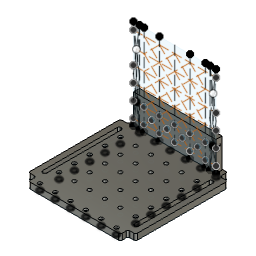
Whole_v2 v3 (Autodesk Fusion 360 design; units mm, degrees)
Autodesk Fusion 360 part; units mm, degrees
(part 1 of 2)
sketch "Sketch1" plane through (0, 0, 0) normal (0, 0, 1) x (1, 0, 0)
  line L0 (73.2, -88.9) -> (-73.2, -88.9)
  line L1 (-88.9, -73.2) -> (-88.9, 73.2)
  line L2 (-73.2, 88.9) -> (73.2, 88.9)
  line L3 (88.9, 73.2) -> (88.9, -73.2)
  line L4 (88.9, -88.9) -> (-88.9, 88.9) construction
  line L5 (-88.9, -88.9) -> (88.9, 88.9) construction
  line L6 (-88.9, 76.2) -> (88.9, 76.2) construction
  line L7 (-88.9, -76.2) -> (88.9, -76.2) construction
  line L8 (-76.2, 88.9) -> (-76.2, -88.9) construction
  line L9 (76.2, 88.9) -> (76.2, -88.9) construction
  line L10 (-76.2, 85.9) -> (-76.2, 79.2)
  line L11 (-85.9, 76.2) -> (-79.2, 76.2)
  line L12 (76.2, 85.9) -> (76.2, 79.2)
  line L13 (79.2, 76.2) -> (85.9, 76.2)
  line L14 (76.2, -76.2) -> (85.9, -76.2)
  line L15 (76.2, -85.9) -> (76.2, -79.2)
  line L16 (-76.2, -85.9) -> (-76.2, -79.2)
  line L17 (-85.9, -76.2) -> (-79.2, -76.2)
  line L18 (-75.85, -65) -> (-76.55, -65)
  line L19 (-79.55, -62) -> (-79.55, 62)
  line L20 (-76.3914, 65) -> (-75.85, 65)
  line L21 (-72.85, 62) -> (-72.85, -62)
  line L22 (-72.85, -65) -> (-79.3874, 61.8456) construction
  line L23 (-79.55, -65) -> (-72.85, 65) construction
  line L24 (76.55, -65) -> (75.85, -65)
  line L25 (72.85, -62) -> (72.85, 62)
  line L26 (75.85, 65) -> (76.55, 65)
  line L27 (79.55, 62) -> (79.55, -62)
  line L28 (79.55, -65) -> (72.85, 65) construction
  line L29 (72.85, -65) -> (79.55, 65) construction
  line L30 (-88.9, 82.55) -> (88.9, 82.55) construction
  line L31 (-63.5, 88.9) -> (-63.5, -88.9) construction
  line L32 (-38.1, 88.9) -> (-38.1, -88.9) construction
  line L33 (-12.7, 88.9) -> (-12.7, -88.9) construction
  line L34 (12.7, 88.9) -> (12.7, -88.9) construction
  line L35 (38.1, 88.9) -> (38.1, -88.9) construction
  line L36 (63.5, 88.9) -> (63.5, -88.9) construction
  line L37 (-88.9, -82.55) -> (88.9, -82.55) construction
  circle A0 centre (-63.5, 82.55) radius 3.1375
  circle A1 centre (-38.1, 82.55) radius 3.1375
  circle A2 centre (-12.7, 82.55) radius 3.1375
  circle A3 centre (12.7, 82.55) radius 3.1375
  circle A4 centre (38.1, 82.55) radius 3.1375
  circle A5 centre (63.5, 82.55) radius 3.1375
  line L38 (-88.9, 0) -> (88.9, 0) construction
  line L39 (-88.9, 50.8) -> (88.9, 50.8) construction
  line L40 (-88.9, 25.4) -> (88.9, 25.4) construction
  line L41 (-88.9, 0) -> (88.9, 0) construction
  line L42 (-88.9, -25.4) -> (88.9, -25.4) construction
  line L43 (-88.9, -50.8) -> (88.9, -50.8) construction
  line L44 (79.2, -76.2) -> (88.9, -76.2) construction
  circle A6 centre (-63.5, -82.55) radius 3.1375
  circle A7 centre (-38.1, -82.55) radius 3.1375
  circle A8 centre (-12.7, -82.55) radius 3.1375
  circle A9 centre (12.7, -82.55) radius 3.1375
  circle A10 centre (38.1, -82.55) radius 3.1375
  circle A11 centre (63.5, -82.55) radius 3.1375
  circle A12 centre (-63.5, 50.8) radius 3.1375
  circle A13 centre (-38.1, 50.8) radius 3.1375
  circle A14 centre (-12.7, 50.8) radius 3.1375
  circle A15 centre (12.7, 50.8) radius 3.1375
  circle A16 centre (38.1, 50.8) radius 3.1375
  circle A17 centre (63.5, 50.8) radius 3.1375
  circle A18 centre (-63.5, 25.4) radius 3.1375
  circle A19 centre (-38.1, 25.4) radius 3.1375
  circle A20 centre (-12.7, 25.4) radius 3.1375
  circle A21 centre (12.7, 25.4) radius 3.1375
  circle A22 centre (38.1, 25.4) radius 3.1375
  circle A23 centre (63.5, 25.4) radius 3.1375
  circle A24 centre (-63.5, 0) radius 3.1375
  circle A25 centre (-38.1, 0) radius 3.1375
  circle A26 centre (-12.7, 0) radius 3.1375
  circle A27 centre (12.7, 0) radius 3.1375
  circle A28 centre (38.1, 0) radius 3.1375
  circle A29 centre (63.5, 0) radius 3.1375
  circle A30 centre (-63.5, -25.4) radius 3.1375
  circle A31 centre (-38.1, -25.4) radius 3.1375
  circle A32 centre (-12.7, -25.4) radius 3.1375
  circle A33 centre (12.7, -25.4) radius 3.1375
  circle A34 centre (38.1, -25.4) radius 3.1375
  circle A35 centre (63.5, -25.4) radius 3.1375
  circle A36 centre (-63.5, -50.8) radius 3.1375
  circle A37 centre (-38.1, -50.8) radius 3.1375
  circle A38 centre (-12.7, -50.8) radius 3.1375
  circle A39 centre (12.7, -50.8) radius 3.1375
  circle A40 centre (38.1, -50.8) radius 3.1375
  circle A41 centre (63.5, -50.8) radius 3.1375
  arc A42 (-73.2, 88.9) -> (-76.2, 85.9) centre (-73.2, 85.9) ccw
  arc A43 (-79.2, 76.2) -> (-76.2, 79.2) centre (-79.2, 79.2) ccw
  arc A44 (-85.9, 76.2) -> (-88.9, 73.2) centre (-85.9, 73.2) ccw
  arc A45 (-72.85, 62) -> (-75.85, 65) centre (-75.85, 62) ccw
  arc A46 (-88.9, -73.2) -> (-85.9, -76.2) centre (-85.9, -73.2) ccw
  arc A47 (-76.2, -79.2) -> (-79.2, -76.2) centre (-79.2, -79.2) ccw
  arc A48 (-76.2, -85.9) -> (-73.2, -88.9) centre (-73.2, -85.9) ccw
  arc A49 (-79.55, -62) -> (-76.55, -65) centre (-76.55, -62) ccw
  arc A50 (-75.85, -65) -> (-72.85, -62) centre (-75.85, -62) ccw
  arc A51 (73.2, -88.9) -> (76.2, -85.9) centre (73.2, -85.9) ccw
  arc A52 (79.2, -76.2) -> (76.2, -79.2) centre (79.2, -79.2) ccw
  arc A53 (85.9, -76.2) -> (88.9, -73.2) centre (85.9, -73.2) ccw
  arc A54 (72.85, -62) -> (75.85, -65) centre (75.85, -62) ccw
  arc A55 (76.55, -65) -> (79.55, -62) centre (76.55, -62) ccw
  arc A56 (76.2, 85.9) -> (73.2, 88.9) centre (73.2, 85.9) ccw
  arc A57 (76.2, 79.2) -> (79.2, 76.2) centre (79.2, 79.2) ccw
  arc A58 (88.9, 73.2) -> (85.9, 76.2) centre (85.9, 73.2) ccw
  arc A59 (75.85, 65) -> (72.85, 62) centre (75.85, 62) ccw
  arc A60 (79.55, 62) -> (76.55, 65) centre (76.55, 62) ccw
  line L45 (-76.3914, 65) -> (-76.55, 65)
  arc A61 (-76.55, 65) -> (-79.55, 62) centre (-76.55, 62) ccw
  point P0 (-79.55, 65)
  point P1 (-76.2, 0)
  point P2 (76.2, 0)
  dimension "d1" = 177.8
  dimension "d2" = 177.8
  dimension "d3" = 12.7
  dimension "d4" = 12.7
  dimension "d5" = 12.7
  dimension "d6" = 12.7
  dimension "d7" = 130
  dimension "d8" = 6.7
  dimension "d9" = 130
  dimension "d10" = 6.7
  dimension "d11" = 6.35
  dimension "d12" = 12.7
  dimension "d13" = 25.4
  dimension "d14" = 25.4
  dimension "d15" = 12.7
  dimension "d16" = 25.4
  dimension "d17" = 25.4
  dimension "d18" = 6.35
  dimension "d19" = 6.275
  dimension "d20" = 6.275
  dimension "d21" = 6.275
  dimension "d22" = 6.275
  dimension "d23" = 6.275
  dimension "d24" = 6.275
  dimension "d25" = 6.275
  dimension "d26" = 6.275
  dimension "d27" = 6.275
  dimension "d28" = 6.275
  dimension "d29" = 6.275
  dimension "d30" = 6.275
  dimension "d31" = 25.4
  dimension "d32" = 25.4
  dimension "d33" = 25.4
  dimension "d34" = 25.4
  dimension "d35" = 25.4
  dimension "d36" = 25.4
  dimension "d37" = 6.275
  dimension "d38" = 6.275
  dimension "d39" = 6.275
  dimension "d40" = 6.275
  dimension "d41" = 6.275
  dimension "d42" = 6.275
  dimension "d43" = 6.275
  dimension "d44" = 6.275
  dimension "d45" = 6.275
  dimension "d46" = 6.275
  dimension "d47" = 6.275
  dimension "d48" = 6.275
  dimension "d49" = 6.275
  dimension "d50" = 6.275
  dimension "d51" = 6.275
  dimension "d52" = 6.275
  dimension "d53" = 6.275
  dimension "d54" = 6.275
  dimension "d55" = 6.275
  dimension "d56" = 6.275
  dimension "d57" = 6.275
  dimension "d58" = 6.275
  dimension "d59" = 6.275
  dimension "d60" = 6.275
  dimension "d61" = 6.275
  dimension "d62" = 6.275
  dimension "d63" = 6.275
  dimension "d64" = 6.275
  dimension "d65" = 6.275
  dimension "d66" = 6.275
  dimension "d67" = 3
  dimension "d68" = 3
  dimension "d69" = 3
  dimension "d71" = 3
  dimension "d72" = 3
  dimension "d73" = 3
  dimension "d74" = 3
  dimension "d75" = 3
  dimension "d76" = 3
  dimension "d77" = 3
  dimension "d78" = 3
  dimension "d79" = 3
  dimension "d80" = 3
  dimension "d81" = 3
  dimension "d82" = 3
  dimension "d83" = 3
  dimension "d84" = 3
  dimension "d85" = 3
  dimension "d86" = 3
  dimension "d87" = 3
  constraint perpendicular L0 L1
  constraint parallel L0 L2
  constraint parallel L1 L3
  constraint horizontal L0
  constraint coincident L4 origin
  constraint coincident L5 origin
  constraint coincident L1 L6.start
  constraint coincident L3 L6.end
  constraint perpendicular L3 L6
  constraint coincident L1 L7.start
  constraint coincident L3 L7.end
  constraint perpendicular L3 L7
  constraint coincident L2 L8.start
  constraint coincident L0 L8.end
  constraint perpendicular L0 L8
  constraint coincident L2 L9.start
  constraint coincident L0 L9.end
  constraint perpendicular L0 L9
  constraint coincident L9 L14.start
  constraint coincident L7 L14.start
  constraint perpendicular L18 L19
  constraint parallel L18 L20
  constraint parallel L19 L21
  constraint horizontal L18
  constraint coincident L22 P1
  constraint coincident L23 P1
  constraint midpoint L8 P1
  constraint perpendicular L24 L25
  constraint parallel L24 L26
  constraint parallel L25 L27
  constraint horizontal L24
  constraint coincident L28 P2
  constraint coincident L29 P2
  constraint midpoint L9 P2
  constraint coincident L1 L30.start
  constraint coincident L3 L30.end
  constraint perpendicular L3 L30
  constraint coincident L2 L31.start
  constraint coincident L0 L31.end
  constraint perpendicular L0 L31
  constraint coincident L2 L32.start
  constraint coincident L0 L32.end
  constraint perpendicular L0 L32
  constraint coincident L2 L33.start
  constraint coincident L0 L33.end
  constraint perpendicular L0 L33
  constraint coincident L2 L34.start
  constraint coincident L0 L34.end
  constraint perpendicular L0 L34
  constraint coincident L2 L35.start
  constraint coincident L0 L35.end
  constraint perpendicular L0 L35
  constraint coincident L2 L36.start
  constraint coincident L0 L36.end
  constraint perpendicular L0 L36
  constraint coincident L1 L37.start
  constraint coincident L3 L37.end
  constraint perpendicular L3 L37
  constraint coincident L30 A0.centre
  constraint coincident L31 A0.centre
  constraint coincident L30 A1.centre
  constraint coincident L32 A1.centre
  constraint coincident L33 A2.centre
  constraint coincident L30 A2.centre
  constraint coincident L30 A3.centre
  constraint coincident L34 A3.centre
  constraint coincident L30 A4.centre
  constraint coincident L35 A4.centre
  constraint coincident L30 A5.centre
  constraint coincident L36 A5.centre
  constraint coincident L1 L39.start
  constraint coincident L3 L39.end
  constraint perpendicular L3 L39
  constraint coincident L1 L40.start
  constraint coincident L3 L40.end
  constraint perpendicular L3 L40
  constraint coincident L1 L38.start
  constraint coincident L3 L38.end
  constraint perpendicular L3 L41
  constraint coincident L1 L42.start
  constraint coincident L3 L42.end
  constraint perpendicular L3 L42
  constraint coincident L1 L43.start
  constraint coincident L3 L43.end
  constraint perpendicular L3 L43
  constraint perpendicular L3 L44
  constraint coincident L37 A6.centre
  constraint coincident L31 A6.centre
  constraint coincident L32 A7.centre
  constraint coincident L37 A7.centre
  constraint coincident L33 A8.centre
  constraint coincident L37 A8.centre
  constraint coincident L34 A9.centre
  constraint coincident L37 A9.centre
  constraint coincident L35 A10.centre
  constraint coincident L37 A10.centre
  constraint coincident L37 A11.centre
  constraint coincident L36 A11.centre
  constraint coincident L39 A12.centre
  constraint coincident L31 A12.centre
  constraint coincident L32 A13.centre
  constraint coincident L39 A13.centre
  constraint coincident L39 A14.centre
  constraint coincident L33 A14.centre
  constraint coincident L34 A15.centre
  constraint coincident L39 A15.centre
  constraint coincident L35 A16.centre
  constraint coincident L39 A16.centre
  constraint coincident L36 A17.centre
  constraint coincident L39 A17.centre
  constraint coincident L40 A18.centre
  constraint coincident L31 A18.centre
  constraint coincident L32 A19.centre
  constraint coincident L40 A19.centre
  constraint coincident L40 A20.centre
  constraint coincident L33 A20.centre
  constraint coincident L34 A21.centre
  constraint coincident L40 A21.centre
  constraint coincident L35 A22.centre
  constraint coincident L40 A22.centre
  constraint coincident L40 A23.centre
  constraint coincident L36 A23.centre
  constraint midpoint L31 A24.centre
  constraint midpoint L32 A25.centre
  constraint midpoint L33 A26.centre
  constraint midpoint L34 A27.centre
  constraint midpoint L35 A28.centre
  constraint midpoint L36 A29.centre
  constraint coincident L42 A30.centre
  constraint coincident L31 A30.centre
  constraint coincident L32 A31.centre
  constraint coincident L42 A31.centre
  constraint coincident L42 A32.centre
  constraint coincident L33 A32.centre
  constraint coincident L42 A33.centre
  constraint coincident L34 A33.centre
  constraint coincident L35 A34.centre
  constraint coincident L42 A34.centre
  constraint coincident L42 A35.centre
  constraint coincident L36 A35.centre
  constraint coincident L31 A36.centre
  constraint coincident L43 A36.centre
  constraint coincident L32 A37.centre
  constraint coincident L43 A37.centre
  constraint coincident L43 A38.centre
  constraint coincident L33 A38.centre
  constraint coincident L43 A39.centre
  constraint coincident L34 A39.centre
  constraint coincident L35 A40.centre
  constraint coincident L43 A40.centre
  constraint coincident L36 A41.centre
  constraint coincident L43 A41.centre
  constraint coincident L8.start L10
  constraint tangent L10 A42
  constraint tangent L2 A42
  constraint tangent L10 A43
  constraint tangent L11 A43
  constraint coincident L6.start L11
  constraint coincident L4.end L1
  constraint tangent L11 A44
  constraint tangent L1 A44
  constraint coincident P0 L20
  constraint coincident P0 L22
  constraint coincident L23.end L21
  constraint coincident L23.end L20
  constraint tangent L21 A45
  constraint tangent L20 A45
  constraint coincident L7.start L17
  constraint coincident L5.start L1
  constraint tangent L17 A46
  constraint tangent L1 A46
  constraint tangent L16 A47
  constraint tangent L17 A47
  constraint coincident L5.start L0
  constraint coincident L8.end L16
  constraint tangent L0 A48
  constraint tangent L16 A48
  constraint coincident L23.start L18
  constraint coincident L23.start L19
  constraint tangent L18 A49
  constraint tangent L19 A49
  constraint coincident L22.start L18
  constraint coincident L22.start L21
  constraint tangent L18 A50
  constraint tangent L21 A50
  constraint coincident L4.start L0
  constraint coincident L9.end L15
  constraint tangent L0 A51
  constraint tangent L15 A51
  constraint coincident L14.start L15
  constraint tangent L15 A52
  constraint tangent L44 A52
  constraint coincident L7.end L14
  constraint coincident L4.start L3
  constraint tangent L14 A53
  constraint tangent L3 A53
  constraint coincident L29.start L24
  constraint coincident L29.start L25
  constraint tangent L24 A54
  constraint tangent L25 A54
  constraint coincident L28.start L24
  constraint coincident L28.start L27
  constraint tangent L24 A55
  constraint tangent L27 A55
  constraint coincident L5.end L2
  constraint coincident L9.start L12
  constraint tangent L2 A56
  constraint tangent L12 A56
  constraint tangent L12 A57
  constraint tangent L13 A57
  constraint coincident L6.end L13
  constraint coincident L5.end L3
  constraint tangent L13 A58
  constraint tangent L3 A58
  constraint coincident L28.end L26
  constraint coincident L28.end L25
  constraint tangent L26 A59
  constraint tangent L25 A59
  constraint coincident L29.end L26
  constraint coincident L29.end L27
  constraint tangent L26 A60
  constraint tangent L27 A60
  constraint coincident P0 L19
  constraint coincident P0 L45
  constraint tangent L19 A61
  constraint tangent L45 A61
  measures "d1" distance of L4.end L5.end
  measures "d2" distance of L5.start L4.end
  measures "d3" distance of L2 L6
  measures "d4" distance of L1 L8
  measures "d5" distance of L3 L9
  measures "d6" distance of L0 L7
  measures "d7" distance of L23.start P0
  measures "d8" distance of P0 L23.end
  measures "d9" distance of L29.start L28.end
  measures "d10" distance of L28.end L29.end
  measures "d11" distance of L2 L30
  measures "d12" distance of L8 L31
  measures "d13" distance of L31 L32
  measures "d14" distance of L32 L33
  measures "d15" distance of L9 L36
  measures "d16" distance of L35 L36
  measures "d17" distance of L34 L35
  measures "d18" distance of L7 L37
  measures "d19" diameter of A0
  measures "d20" diameter of A1
  measures "d21" diameter of A2
  measures "d22" diameter of A3
  measures "d23" diameter of A4
  measures "d24" diameter of A5
  measures "d25" diameter of A6
  measures "d26" diameter of A7
  measures "d27" diameter of A8
  measures "d28" diameter of A9
  measures "d29" diameter of A10
  measures "d30" diameter of A11
  measures "d31" distance of L6 L39
  measures "d32" distance of L39 L40
  measures "d33" distance of L40 L41
  measures "d34" distance of L38 L42
  measures "d35" distance of L42 L43
  measures "d36" distance of L43 L44
  measures "d37" diameter of A12
  measures "d38" diameter of A13
  measures "d39" diameter of A14
  measures "d40" diameter of A15
  measures "d41" diameter of A16
  measures "d42" diameter of A17
  measures "d43" diameter of A18
  measures "d44" diameter of A19
  measures "d45" diameter of A20
  measures "d46" diameter of A21
  measures "d47" diameter of A22
  measures "d48" diameter of A23
  measures "d49" diameter of A24
  measures "d50" diameter of A25
  measures "d51" diameter of A26
  measures "d52" diameter of A27
  measures "d53" diameter of A28
  measures "d54" diameter of A29
  measures "d55" diameter of A30
  measures "d56" diameter of A31
  measures "d57" diameter of A32
  measures "d58" diameter of A33
  measures "d59" diameter of A34
  measures "d60" diameter of A35
  measures "d61" diameter of A36
  measures "d62" diameter of A37
  measures "d63" diameter of A38
  measures "d64" diameter of A39
  measures "d65" diameter of A40
  measures "d66" diameter of A41
  measures "d67" radius of A42
  measures "d68" radius of A43
  measures "d69" radius of A44
  measures "d71" radius of A45
  measures "d72" radius of A46
  measures "d73" radius of A47
  measures "d74" radius of A48
  measures "d75" radius of A49
  measures "d76" radius of A50
  measures "d77" radius of A51
  measures "d78" radius of A52
  measures "d79" radius of A53
  measures "d80" radius of A54
  measures "d81" radius of A55
  measures "d82" radius of A56
  measures "d83" radius of A57
  measures "d84" radius of A58
  measures "d85" radius of A59
  measures "d86" radius of A60
  measures "d87" radius of A61
extrude "Extrude1" add sketch "Sketch1" along normal blind 10 makes body 1
sketch "Sketch1 (2)" plane through (0, 0, 10) normal (0, 0, 1) x (-1, 0, 0) in component "Back"
  circle A0 centre (-12.7, 25.4) radius 3.1375
  circle A1 centre (12.7, 25.4) radius 3.1375
  line L0 (76.55, -65) -> (75.85, -65)
  arc A2 (72.85, -62) -> (75.85, -65) centre (75.85, -62) ccw
  line L1 (72.85, -62) -> (72.85, 62)
  arc A3 (75.85, 65) -> (72.85, 62) centre (75.85, 62) ccw
  line L2 (75.85, 65) -> (76.55, 65)
  arc A4 (79.55, 62) -> (76.55, 65) centre (76.55, 62) ccw
  line L3 (79.55, 62) -> (79.55, -62)
  arc A5 (76.55, -65) -> (79.55, -62) centre (76.55, -62) ccw
  arc A6 (-76.55, 65) -> (-79.55, 62) centre (-76.55, 62) ccw
  line L4 (-76.55, 65) -> (-75.85, 65)
  arc A7 (-72.85, 62) -> (-75.85, 65) centre (-75.85, 62) ccw
  line L5 (-72.85, 62) -> (-72.85, -62)
  arc A8 (-75.85, -65) -> (-72.85, -62) centre (-75.85, -62) ccw
  line L6 (-75.85, -65) -> (-76.55, -65)
  arc A9 (-79.55, -62) -> (-76.55, -65) centre (-76.55, -62) ccw
  line L7 (-79.55, -62) -> (-79.55, 62)
  circle A10 centre (-63.5, 50.8) radius 3.1375
  circle A11 centre (-38.1, 50.8) radius 3.1375
  circle A12 centre (-12.7, 50.8) radius 3.1375
  circle A13 centre (12.7, 50.8) radius 3.1375
  circle A14 centre (38.1, 50.8) radius 3.1375
  circle A15 centre (63.5, 50.8) radius 3.1375
  circle A16 centre (-63.5, 25.4) radius 3.1375
  circle A17 centre (-38.1, 25.4) radius 3.1375
  circle A18 centre (12.7, -50.8) radius 3.1375
  circle A19 centre (-12.7, -50.8) radius 3.1375
  circle A20 centre (-38.1, -50.8) radius 3.1375
  circle A21 centre (-63.5, -50.8) radius 3.1375
  circle A22 centre (63.5, -25.4) radius 3.1375
  circle A23 centre (38.1, -25.4) radius 3.1375
  circle A24 centre (12.7, -25.4) radius 3.1375
  circle A25 centre (-63.5, 0) radius 3.1375
  circle A26 centre (63.5, 25.4) radius 3.1375
  circle A27 centre (38.1, 25.4) radius 3.1375
  circle A28 centre (38.1, -50.8) radius 3.1375
  circle A29 centre (63.5, -50.8) radius 3.1375
  circle A30 centre (-63.5, 82.55) radius 3.1375
  circle A31 centre (-38.1, 82.55) radius 3.1375
  circle A32 centre (-12.7, 82.55) radius 3.1375
  circle A33 centre (12.7, 82.55) radius 3.1375
  circle A34 centre (38.1, 82.55) radius 3.1375
  circle A35 centre (63.5, 82.55) radius 3.1375
  circle A36 centre (-63.5, -82.55) radius 3.1375
  circle A37 centre (-38.1, -82.55) radius 3.1375
  circle A38 centre (-12.7, -82.55) radius 3.1375
  circle A39 centre (12.7, -82.55) radius 3.1375
  circle A40 centre (38.1, -82.55) radius 3.1375
  circle A41 centre (63.5, -82.55) radius 3.1375
  circle A42 centre (-63.5, -25.4) radius 3.1375
  circle A43 centre (-12.7, -25.4) radius 3.1375
  circle A44 centre (-38.1, 0) radius 3.1375
  circle A45 centre (38.1, 0) radius 3.1375
  circle A46 centre (-12.7, 0) radius 3.1375
  circle A47 centre (-38.1, -25.4) radius 3.1375
  circle A48 centre (63.5, 0) radius 3.1375
  circle A49 centre (12.7, 0) radius 3.1375
  line L8 (-79.2, 76.2) -> (-85.9, 76.2)
  arc A50 (-85.9, 76.2) -> (-88.9, 73.2) centre (-85.9, 73.2) ccw
  line L9 (-88.9, 73.2) -> (-88.9, -73.2)
  arc A51 (-88.9, -73.2) -> (-85.9, -76.2) centre (-85.9, -73.2) ccw
  line L10 (-85.9, -76.2) -> (-79.2, -76.2)
  arc A52 (-76.2, -79.2) -> (-79.2, -76.2) centre (-79.2, -79.2) ccw
  line L11 (-76.2, -79.2) -> (-76.2, -85.9)
  arc A53 (-76.2, -85.9) -> (-73.2, -88.9) centre (-73.2, -85.9) ccw
  line L12 (-73.2, -88.9) -> (73.2, -88.9)
  arc A54 (73.2, -88.9) -> (76.2, -85.9) centre (73.2, -85.9) ccw
  line L13 (76.2, -85.9) -> (76.2, -79.2)
  arc A55 (79.2, -76.2) -> (76.2, -79.2) centre (79.2, -79.2) ccw
  line L14 (79.2, -76.2) -> (85.9, -76.2)
  arc A56 (85.9, -76.2) -> (88.9, -73.2) centre (85.9, -73.2) ccw
  line L15 (88.9, -73.2) -> (88.9, 73.2)
  arc A57 (88.9, 73.2) -> (85.9, 76.2) centre (85.9, 73.2) ccw
  line L16 (85.9, 76.2) -> (79.2, 76.2)
  arc A58 (76.2, 79.2) -> (79.2, 76.2) centre (79.2, 79.2) ccw
  line L17 (76.2, 79.2) -> (76.2, 85.9)
  arc A59 (76.2, 85.9) -> (73.2, 88.9) centre (73.2, 85.9) ccw
  line L18 (73.2, 88.9) -> (-73.2, 88.9)
  arc A60 (-73.2, 88.9) -> (-76.2, 85.9) centre (-73.2, 85.9) ccw
  line L19 (-76.2, 85.9) -> (-76.2, 79.2)
  arc A61 (-79.2, 76.2) -> (-76.2, 79.2) centre (-79.2, 79.2) ccw
  line L20 (76.2, -75.4206) -> (76.2, -89.5685) construction
  line L21 (66.5936, -88.9) -> (82, -88.9) construction
  line L22 (-76.2, -73.4985) -> (-76.2, -92.9771) construction
  line L23 (-61.7398, -88.9) -> (-86.4306, -88.9) construction
  line L24 (-84.2129, -76.2) -> (-69, -76.2) construction
  line L25 (83.8181, -76.2) -> (64, -76.2) construction
  line L26 (63.5, -82.55) -> (-63.5, -82.55) construction
  line L27 (63.5, -82.55) -> (63.5, -88.9) construction
  line L28 (-63.5, -82.55) -> (-63.5, -88.9) construction
  line L29 (0, -88.9) -> (0, -50) construction
  line L30 (68.5, -77.55) -> (-68.5, -77.55)
  line L31 (-68.5, -77.55) -> (-68.5, -87.55)
  line L32 (-68.5, -87.55) -> (68.5, -87.55)
  line L33 (68.5, -87.55) -> (68.5, -77.55)
  line L34 (68.5, -77.55) -> (-68.5, -87.55) construction
  line L35 (-68.5, -77.55) -> (68.5, -87.55) construction
  point P0 (0, -82.55)
  dimension "d90" = 137
  dimension "d91" = 10
  constraint coincident L13 L20.start
  constraint parallel L13 L20
  constraint coincident L12 L21.start
  constraint parallel L12 L21
  constraint coincident L11 L22.start
  constraint parallel L11 L22
  constraint coincident L12 L23.start
  constraint perpendicular L22 L23
  constraint coincident L10 L24.start
  constraint perpendicular L22 L24
  constraint coincident L14 L25.start
  constraint perpendicular L13 L25
  constraint coincident A41.centre L26.start
  constraint coincident A36.centre L26.end
  constraint coincident L12 L27.end
  constraint perpendicular L12 L27
  constraint vertical L28
  constraint coincident L23 L28.end
  constraint midpoint L12 L29.start
  constraint perpendicular L12 L29
  constraint perpendicular L30 L31
  constraint parallel L30 L32
  constraint parallel L31 L33
  constraint horizontal L30
  constraint coincident L34 P0
  constraint coincident L35 P0
  constraint midpoint L26 P0
  measures "d90" distance of L31.end L32.end
  measures "d91" distance of L30.end L31.end
extrude "Extrude1'" add sketch "Sketch1 (2)" along normal blind 150 separate body contours A36 | A37 | A38 | A39 | A40 | A41 | L30 L31 L32 L33 makes body 2 in component "Back"
sketch "Sketch2" plane through (0, 0, 10) normal (0, 0, -1) x (1, 0, 0) in component "Back"
  line L0 (-68.5, -77.55) -> (-68.5, -87.55)
  line L1 (-68.5, -87.55) -> (68.5, -87.55)
  line L2 (68.5, -87.55) -> (68.5, -77.55)
  line L3 (68.5, -77.55) -> (-68.5, -77.55)
  line L4 (-68.5, -82.55) -> (68.5, -82.55) construction
  line L5 (-12.7, -77.55) -> (-12.7, -87.55) construction
  line L6 (12.7, -77.55) -> (12.7, -87.55) construction
  line L7 (38.1, -77.55) -> (38.1, -87.55) construction
  line L8 (63.5, -77.55) -> (63.5, -87.55) construction
  line L9 (-63.5, -77.55) -> (-63.5, -87.55) construction
  line L10 (-38.1, -77.55) -> (-38.1, -87.55) construction
  circle A0 centre (-63.5, -82.55) radius 3.1375
  circle A1 centre (-38.1, -82.55) radius 3.1375
  circle A2 centre (-12.7, -82.55) radius 3.1375
  circle A3 centre (12.7, -82.55) radius 3.1375
  circle A4 centre (38.1, -82.55) radius 3.1375
  circle A5 centre (63.5, -82.55) radius 3.1375
  dimension "d94" = 5
  dimension "d95" = 25.4
  dimension "d96" = 25.4
  dimension "d97" = 25.4
  dimension "d98" = 25.4
  dimension "d99" = 25.4
  dimension "d100" = 6.275
  dimension "d101" = 6.275
  dimension "d102" = 6.275
  dimension "d103" = 6.275
  dimension "d104" = 6.275
  dimension "d105" = 6.275
  constraint midpoint L0 L4.start
  constraint midpoint L2 L4.end
  constraint coincident L3 L5.start
  constraint coincident L1 L5.end
  constraint perpendicular L1 L5
  constraint coincident L3 L6.start
  constraint coincident L1 L6.end
  constraint perpendicular L1 L6
  constraint coincident L3 L7.start
  constraint coincident L1 L7.end
  constraint perpendicular L1 L7
  constraint coincident L3 L8.start
  constraint coincident L1 L8.end
  constraint perpendicular L1 L8
  constraint coincident L3 L9.start
  constraint coincident L1 L9.end
  constraint perpendicular L1 L9
  constraint coincident L3 L10.start
  constraint coincident L1 L10.end
  constraint perpendicular L1 L10
  constraint midpoint L9 A0.centre
  constraint midpoint L10 A1.centre
  constraint midpoint L5 A2.centre
  constraint midpoint L6 A3.centre
  constraint midpoint L7 A4.centre
  constraint midpoint L8 A5.centre
  measures "d94" distance of L2 L8
  measures "d95" distance of L7 L8
  measures "d96" distance of L6 L7
  measures "d97" distance of L5 L6
  measures "d98" distance of L5 L10
  measures "d99" distance of L9 L10
  measures "d100" diameter of A0
  measures "d101" diameter of A1
  measures "d102" diameter of A2
  measures "d103" diameter of A3
  measures "d104" diameter of A4
  measures "d105" diameter of A5
extrude "Extrude2" cut sketch "Sketch2" against normal blind 25 contours A0 | A1 | A2 | A3 | A4 | A5 bodies 2 in component "Back"
sketch "Sketch1 (3)" plane through (0, 0, 10) normal (0, 0, 1) x (-1, 0, 0) in component "Side"
  circle A0 centre (-12.7, 25.4) radius 3.1375
  circle A1 centre (12.7, 25.4) radius 3.1375
  line L0 (76.55, -65) -> (75.85, -65)
  arc A2 (72.85, -62) -> (75.85, -65) centre (75.85, -62) ccw
  line L1 (72.85, -62) -> (72.85, 62)
  arc A3 (75.85, 65) -> (72.85, 62) centre (75.85, 62) ccw
  line L2 (75.85, 65) -> (76.55, 65)
  arc A4 (79.55, 62) -> (76.55, 65) centre (76.55, 62) ccw
  line L3 (79.55, 62) -> (79.55, -62)
  arc A5 (76.55, -65) -> (79.55, -62) centre (76.55, -62) ccw
  arc A6 (-76.55, 65) -> (-79.55, 62) centre (-76.55, 62) ccw
  line L4 (-76.55, 65) -> (-75.85, 65)
  arc A7 (-72.85, 62) -> (-75.85, 65) centre (-75.85, 62) ccw
  line L5 (-72.85, 62) -> (-72.85, -62)
  arc A8 (-75.85, -65) -> (-72.85, -62) centre (-75.85, -62) ccw
  line L6 (-75.85, -65) -> (-76.55, -65)
  arc A9 (-79.55, -62) -> (-76.55, -65) centre (-76.55, -62) ccw
  line L7 (-79.55, -62) -> (-79.55, 62)
  circle A10 centre (-63.5, 50.8) radius 3.1375
  circle A11 centre (-38.1, 50.8) radius 3.1375
  circle A12 centre (-12.7, 50.8) radius 3.1375
  circle A13 centre (12.7, 50.8) radius 3.1375
  circle A14 centre (38.1, 50.8) radius 3.1375
  circle A15 centre (63.5, 50.8) radius 3.1375
  circle A16 centre (-63.5, 25.4) radius 3.1375
  circle A17 centre (-38.1, 25.4) radius 3.1375
  circle A18 centre (12.7, -50.8) radius 3.1375
  circle A19 centre (-12.7, -50.8) radius 3.1375
  circle A20 centre (-38.1, -50.8) radius 3.1375
  circle A21 centre (-63.5, -50.8) radius 3.1375
  circle A22 centre (63.5, -25.4) radius 3.1375
  circle A23 centre (38.1, -25.4) radius 3.1375
  circle A24 centre (12.7, -25.4) radius 3.1375
  circle A25 centre (-63.5, 0) radius 3.1375
  circle A26 centre (63.5, 25.4) radius 3.1375
  circle A27 centre (38.1, 25.4) radius 3.1375
  circle A28 centre (38.1, -50.8) radius 3.1375
  circle A29 centre (63.5, -50.8) radius 3.1375
  circle A30 centre (-63.5, 82.55) radius 3.1375
  circle A31 centre (-38.1, 82.55) radius 3.1375
  circle A32 centre (-12.7, 82.55) radius 3.1375
  circle A33 centre (12.7, 82.55) radius 3.1375
  circle A34 centre (38.1, 82.55) radius 3.1375
  circle A35 centre (63.5, 82.55) radius 3.1375
  circle A36 centre (-63.5, -82.55) radius 3.1375
  circle A37 centre (-38.1, -82.55) radius 3.1375
  circle A38 centre (-12.7, -82.55) radius 3.1375
  circle A39 centre (12.7, -82.55) radius 3.1375
  circle A40 centre (38.1, -82.55) radius 3.1375
  circle A41 centre (63.5, -82.55) radius 3.1375
  circle A42 centre (-63.5, -25.4) radius 3.1375
  circle A43 centre (-12.7, -25.4) radius 3.1375
  circle A44 centre (-38.1, 0) radius 3.1375
  circle A45 centre (38.1, 0) radius 3.1375
  circle A46 centre (-12.7, 0) radius 3.1375
  circle A47 centre (-38.1, -25.4) radius 3.1375
  circle A48 centre (63.5, 0) radius 3.1375
  circle A49 centre (12.7, 0) radius 3.1375
  line L8 (-79.2, 76.2) -> (-85.9, 76.2)
  arc A50 (-85.9, 76.2) -> (-88.9, 73.2) centre (-85.9, 73.2) ccw
  line L9 (-88.9, 73.2) -> (-88.9, -73.2)
  arc A51 (-88.9, -73.2) -> (-85.9, -76.2) centre (-85.9, -73.2) ccw
  line L10 (-85.9, -76.2) -> (-79.2, -76.2)
  arc A52 (-76.2, -79.2) -> (-79.2, -76.2) centre (-79.2, -79.2) ccw
  line L11 (-76.2, -79.2) -> (-76.2, -85.9)
  arc A53 (-76.2, -85.9) -> (-73.2, -88.9) centre (-73.2, -85.9) ccw
  line L12 (-73.2, -88.9) -> (73.2, -88.9)
  arc A54 (73.2, -88.9) -> (76.2, -85.9) centre (73.2, -85.9) ccw
  line L13 (76.2, -85.9) -> (76.2, -79.2)
  arc A55 (79.2, -76.2) -> (76.2, -79.2) centre (79.2, -79.2) ccw
  line L14 (79.2, -76.2) -> (85.9, -76.2)
  arc A56 (85.9, -76.2) -> (88.9, -73.2) centre (85.9, -73.2) ccw
  line L15 (88.9, -73.2) -> (88.9, 73.2)
  arc A57 (88.9, 73.2) -> (85.9, 76.2) centre (85.9, 73.2) ccw
  line L16 (85.9, 76.2) -> (79.2, 76.2)
  arc A58 (76.2, 79.2) -> (79.2, 76.2) centre (79.2, 79.2) ccw
  line L17 (76.2, 79.2) -> (76.2, 85.9)
  arc A59 (76.2, 85.9) -> (73.2, 88.9) centre (73.2, 85.9) ccw
  line L18 (73.2, 88.9) -> (-73.2, 88.9)
  arc A60 (-73.2, 88.9) -> (-76.2, 85.9) centre (-73.2, 85.9) ccw
  line L19 (-76.2, 85.9) -> (-76.2, 79.2)
  arc A61 (-79.2, 76.2) -> (-76.2, 79.2) centre (-79.2, 79.2) ccw
  line L20 (63.5, -82.55) -> (63.5, 63) construction
  line L21 (-63.5, -82.55) -> (-63.5, 64.4003) construction
  line L22 (58.5, 63) -> (58.5, -80) construction
  line L23 (-58.5, 64.4003) -> (-58.5, -80) construction
  line L24 (-68.5, 64.1213) -> (-68.5, -80) construction
  line L25 (68.5, 63) -> (68.5, -80) construction
  line L26 (69.9113, -82.55) -> (-72.5639, -82.55) construction
  line L27 (72.6784, -77.55) -> (-100, -77.55) construction
  line L28 (68.5, 55.8) -> (-68.5, 55.8) construction
  line L29 (12.7, 50.8) -> (-12.7, 50.8) construction
  line L30 (58.5, -77.55) -> (68.5, -77.55)
  line L31 (68.5, -77.55) -> (68.5, 55.8)
  line L32 (68.5, 55.8) -> (58.5, 55.8)
  line L33 (58.5, 55.8) -> (58.5, -77.55)
  dimension "d108" = 5
  dimension "d109" = 5
  dimension "d110" = 5
  dimension "d111" = 5
  dimension "d112" = 142.4753
  dimension "d113" = 5
  dimension "d114" = 5
  constraint coincident A41.centre L20.start
  constraint vertical L20
  constraint coincident A36.centre L21.start
  constraint vertical L21
  constraint parallel L5 L22
  constraint parallel L21 L23
  constraint parallel L5 L24
  constraint parallel L20 L25
  constraint perpendicular L11 L26
  constraint perpendicular L11 L27
  constraint coincident L25 L28.start
  constraint coincident L24 L28.end
  constraint perpendicular L24 L28
  constraint coincident A13.centre L29.start
  constraint coincident A12.centre L29.end
  constraint horizontal L30
  constraint vertical L31
  constraint horizontal L32
  constraint vertical L33
  constraint coincident L27 L30.start
  constraint coincident L22 L30.start
  measures "d108" distance of L20 L25
  measures "d109" distance of L20 L22
  measures "d110" distance of L21 L24
  measures "d111" distance of L21 L23
  measures "d112" distance of L26.start L26.end
  measures "d113" distance of L26 L27
  measures "d114" distance of L28 L29
extrude "Extrude1''" add sketch "Sketch1 (3)" along normal blind 150 separate body contours A15 | A22 | A26 | A29 | A48 | L30 L31 L32 L33 makes body 3 in component "Side"
sketch "Sketch2 (2)" plane through (0, 0, 10) normal (0, 0, -1) x (1, 0, 0) in component "Side"
  line L0 (-58.5, -77.55) -> (-58.5, 55.8)
  line L1 (-58.5, 55.8) -> (-68.5, 55.8)
  line L2 (-68.5, 55.8) -> (-68.5, -77.55)
  line L3 (-68.5, -77.55) -> (-58.5, -77.55)
  line L4 (-63.5, 55.8) -> (-63.5, -77.55) construction
  line L5 (-68.5, 50.8) -> (-58.5, 50.8) construction
  line L6 (-68.5, 25.4) -> (-58.5, 25.4) construction
  circle A0 centre (-63.5, 50.8) radius 3.1375
  circle A1 centre (-63.5, 25.4) radius 3.1375
  dimension "d117" = 5
  dimension "d118" = 25.4
  dimension "d119" = 6.275
  dimension "d120" = 6.275
  constraint midpoint L1 L4.start
  constraint midpoint L3 L4.end
  constraint coincident L2 L5.start
  constraint coincident L0 L5.end
  constraint perpendicular L0 L5
  constraint coincident L2 L6.start
  constraint coincident L0 L6.end
  constraint perpendicular L0 L6
  constraint midpoint L5 A0.centre
  constraint midpoint L6 A1.centre
  measures "d117" distance of L1 L5
  measures "d118" distance of L5 L6
  measures "d119" diameter of A0
  measures "d120" diameter of A1
extrude "Extrude2'" cut sketch "Sketch2 (2)" against normal up to surface (150 mm away) contours A0 | A1 bodies 3 in component "Side"
sketch "Sketch3" plane through (-68.5, 0, 0) normal (-1, 0, 0) x (0, -1, 0) in component "Side"
  line L0 (-77.55, 10) -> (55.8, 10)
  line L1 (55.8, 10) -> (55.8, 160)
  line L2 (55.8, 160) -> (-77.55, 160)
  line L3 (-77.55, 160) -> (-77.55, 10)
  line L4 (-77.55, 20) -> (52.8, 20) construction
  line L5 (20.4, 160) -> (20.4, 10) construction
  line L6 (55.8, 90) -> (-52.55, 90) construction
  line L7 (-67.55, 157) -> (-67.55, 10) construction
  line L8 (55.8, 95) -> (-77.55, 95) construction
  line L9 (55.8, 115) -> (-77.55, 115) construction
  line L10 (-0.0002, 160) -> (-0.0002, 10) construction
  line L11 (14.9998, 160) -> (14.9998, 10) construction
  line L12 (-15.0002, 160) -> (-15.0002, 10) construction
  line L13 (-67.55, 160) -> (-67.55, 105)
  line L14 (-67.55, 90) -> (-20.0002, 90)
  line L15 (-15.0002, 95) -> (-15.0002, 112)
  line L16 (-12.0002, 115) -> (11.9998, 115)
  line L17 (14.9998, 112) -> (14.9998, 93)
  line L18 (17.9998, 90) -> (18.4, 90)
  line L19 (20.4, 88) -> (20.4, 35)
  line L20 (35.4, 20) -> (55.8, 20)
  line L21 (14.9998, 115) -> (-15.0002, 95) construction
  line L22 (-15.0002, 115) -> (14.9998, 95) construction
  line L23 (-0.0002, 95) -> (-0.0002, 95)
  line L24 (-5.0002, 100) -> (-5.0002, 115)
  line L25 (-5.0002, 115) -> (4.9998, 115)
  line L26 (4.9998, 115) -> (4.9998, 100)
  line L27 (4.9998, 95) -> (-5.0002, 115) construction
  line L28 (-5.0002, 95) -> (4.9998, 115) construction
  line L29 (-77.55, 160) -> (-70.55, 160)
  line L30 (55.8, 10) -> (55.8, 17)
  arc A0 (-67.55, 157) -> (-70.55, 160) centre (-70.55, 157) ccw
  arc A1 (-67.55, 105) -> (-52.55, 90) centre (-52.55, 105) ccw
  arc A2 (-20.0002, 90) -> (-15.0002, 95) centre (-20.0002, 95) ccw
  arc A3 (-12.0002, 115) -> (-15.0002, 112) centre (-12.0002, 112) ccw
  arc A4 (-5.0002, 100) -> (-0.0002, 95) centre (-0.0002, 100) ccw
  arc A5 (-0.0002, 95) -> (4.9998, 100) centre (-0.0002, 100) ccw
  arc A6 (14.9998, 112) -> (11.9998, 115) centre (11.9998, 112) ccw
  arc A7 (14.9998, 93) -> (17.9998, 90) centre (17.9998, 93) ccw
  arc A8 (20.4, 88) -> (18.4, 90) centre (18.4, 88) ccw
  arc A9 (55.8, 17) -> (52.8, 20) centre (52.8, 17) ccw
  arc A10 (20.4, 35) -> (35.4, 20) centre (35.4, 35) ccw
  point P0 (-0.0002, 105)
  dimension "d123" = 10
  dimension "d124" = 35.4
  dimension "d125" = 80
  dimension "d126" = 10
  dimension "d127" = 5
  dimension "d128" = 20
  dimension "d129" = 15
  dimension "d130" = 15
  dimension "d131" = 10
  dimension "d132" = 3
  dimension "d133" = 15
  dimension "d134" = 5
  dimension "d135" = 3
  dimension "d136" = 5
  dimension "d137" = 5
  dimension "d138" = 3
  dimension "d139" = 3
  dimension "d140" = 2
  dimension "d141" = 3
  dimension "d142" = 15
  constraint coincident L3 L4.start
  constraint coincident L1 L20.end
  constraint perpendicular L1 L4
  constraint coincident L2 L5.start
  constraint coincident L0 L5.end
  constraint perpendicular L0 L5
  constraint coincident L1 L6.start
  constraint perpendicular L3 L6
  constraint coincident L2 L13.start
  constraint coincident L0 L7.end
  constraint perpendicular L0 L7
  constraint coincident L1 L8.start
  constraint coincident L3 L8.end
  constraint perpendicular L3 L8
  constraint coincident L1 L9.start
  constraint coincident L3 L9.end
  constraint perpendicular L3 L9
  constraint coincident L2 L10.start
  constraint coincident L0 L10.end
  constraint perpendicular L0 L10
  constraint coincident L2 L11.start
  constraint coincident L0 L11.end
  constraint perpendicular L0 L11
  constraint coincident L2 L12.start
  constraint coincident L0 L12.end
  constraint perpendicular L0 L12
  constraint coincident L7 L14.start
  constraint coincident L6 L14.start
  constraint coincident L9 L22.start
  constraint coincident L12 L22.start
  constraint coincident L9 L21.start
  constraint coincident L11 L21.start
  constraint coincident L8 L15.start
  constraint coincident L12 L15.start
  constraint coincident L8 L22.end
  constraint coincident L17 L22.end
  constraint parallel L24 L26
  constraint coincident L27 P0
  constraint coincident L28 P0
  constraint midpoint L22 P0
  constraint coincident L2.end L3.start
  constraint coincident L0.end L1.start
  constraint coincident L13.start L29
  constraint coincident L13.start L7
  constraint tangent L29 A0
  constraint tangent L7 A0
  constraint coincident L14.start L13
  constraint tangent L13 A1
  constraint tangent L6 A1
  constraint tangent L14 A2
  constraint tangent L15 A2
  constraint coincident L22.start L16
  constraint coincident L22.start L15
  constraint tangent L16 A3
  constraint tangent L15 A3
  constraint coincident L28.start L24
  constraint tangent L24 A4
  constraint coincident L27.start L23
  constraint coincident L27.start L26
  constraint tangent L26 A5
  constraint coincident L21.start L17
  constraint coincident L21.start L16
  constraint tangent L17 A6
  constraint tangent L16 A6
  constraint tangent L17 A7
  constraint tangent L18 A7
  constraint tangent L19 A8
  constraint tangent L18 A8
  constraint coincident L20.end L30
  constraint coincident L20.end L4
  constraint tangent L30 A9
  constraint tangent L4 A9
  constraint tangent L20 A10
  constraint tangent L19 A10
  measures "d123" distance of L0 L4
  measures "d124" distance of L1 L5
  measures "d125" distance of L0 L6
  measures "d126" distance of L3 L7
  measures "d127" distance of L6 L8
  measures "d128" distance of L8 L9
  measures "d129" distance of L10 L11
  measures "d130" distance of L10 L12
  measures "d131" distance of L24.end L25.end
  measures "d132" radius of A0
  measures "d133" radius of A1
  measures "d134" radius of A2
  measures "d135" radius of A3
  measures "d136" radius of A4
  measures "d137" radius of A5
  measures "d138" radius of A6
  measures "d139" radius of A7
  measures "d140" radius of A8
  measures "d141" radius of A9
  measures "d142" radius of A10
extrude "Extrude3" cut sketch "Sketch3" against normal up to surface (10 mm away) contours L1 L2 L13 L14 L15 L16 L17 L18 L19 L20 L25 A1 A2 A3 A6 A7 A8 A10 | L16 L24 L25 L26 A4 A5 bodies 3 in component "Side"
sketch "Sketch4" plane through (0, 0, 115) normal (0, 0, 1) x (-1, 0, 0) in component "Side"
  line L0 (58.5, 11.9998) -> (58.5, 4.9998)
  line L1 (58.5, 4.9998) -> (68.5, 4.9998)
  line L2 (68.5, 4.9998) -> (68.5, 11.9998)
  line L3 (68.5, 11.9998) -> (58.5, 11.9998)
  line L4 (68.5, 11.9998) -> (63.5, 4.9998) construction
  line L5 (63.5, 4.9998) -> (58.5, 11.9998) construction
  line L6 (59.5, 11.9998) -> (59.5, -15.0404) construction
  line L7 (63.5, 4.9998) -> (63.5, 11.9998) construction
  line L8 (67.5, 11.9998) -> (67.5, 4.9998) construction
  line L9 (67.5, 11.9998) -> (59.5, 11.9998)
  line L10 (59.5, 11.9998) -> (59.5, -12.0002)
  line L11 (59.5, -12.0002) -> (67.5, -12.0002)
  line L12 (67.5, -12.0002) -> (67.5, 11.9998)
  dimension "d145" = 4
  dimension "d147" = 8
  dimension "d148" = 24
  constraint coincident L2.end L3.start
  constraint midpoint L1 L4.end
  constraint coincident L0.start L3.end
  constraint coincident L3 L6.start
  constraint perpendicular L3 L6
  constraint midpoint L3 L7.end
  constraint coincident L3 L8.start
  constraint coincident L1 L8.end
  constraint perpendicular L1 L8
  constraint horizontal L9
  constraint vertical L10
  constraint horizontal L11
  constraint vertical L12
  measures "d145" distance of L6 L7
  measures "d147" distance of L6 L8
  measures "d148" distance of L8.start L11.end
extrude "Extrude4" cut sketch "Sketch4" against normal up to surface (25 mm away) contours L1 L3 L9 L10 L12 | L1 L10 L11 L12 bodies 3 in component "Side"